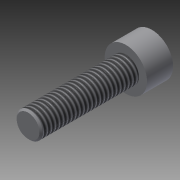
# Autodesk Inventor part: 8x30mmSHCS
Saved by Autodesk Inventor 2014 SP1 (Build 180222100, 222)
## iProperties
Created: 2013-12-15
Part Number: 8x30mmSHCS
Material: Stainless Steel
Document SubType Name: Modeling
Designer: Jack
Density: 8.08 g/cm^3
Appearance: Semi-Polished
Author: Jack
Autodesk Inventor part; units mm, degrees
ref_plane "YZ Plane" through (0, 0, 0) normal (1, 0, 0) x (0, 1, 0)
ref_plane "XZ Plane" through (0, 0, 0) normal (0, 1, 0) x (-1, 0, 0)
ref_plane "XY Plane" through (0, 0, 0) normal (0, 0, 1) x (1, 0, 0)
sketch "Sketch1" plane through (0, 0, 0) normal (0, 1, 0) x (-1, 0, 0)
  circle A0 centre (0, 0) radius 4
  dimension "d0" = 8
  constraints: 1 centre point, 1 coincident
  measures "d0" diameter of A0
extrude "Extrusion1" add sketch "Sketch1" along normal blind 30
sketch "Sketch2" plane through (0, 30, 0) normal (0, 1, 0) x (1, 0, 0)
  circle A0 centre (0, 0) radius 4 projected
  circle A1 centre (0, 0) radius 6.5
  dimension "d3" = 13
  constraints: 1 centre point, 1 coincident
  measures "d3" diameter of A1
extrude "Extrusion2" add sketch "Sketch2" along normal blind 8 contours A0 | A1
sketch "Sketch3" plane through (0, 38, 0) normal (0, 1, 0) x (1, 0, 0)
  circle A0 centre (0, 0) radius 6.5 projected
  line L0 (0, 3.4641) -> (3, 1.7321)
  line L1 (3, 1.7321) -> (3, -1.7321)
  line L2 (3, -1.7321) -> (0, -3.4641)
  line L3 (0, -3.4641) -> (-3, -1.7321)
  line L4 (-3, -1.7321) -> (-3, 1.7321)
  line L5 (-3, 1.7321) -> (0, 3.4641)
  dimension "d6" = 6
  constraints: 12 end point, 1 coincident, 1 vertical, 13 other
  measures "d6" distance between parallel lines of L1 L4
extrude "Extrusion3" cut sketch "Sketch3" against normal blind 6 contours L0 L1 L2 L3 L4 L5
thread "Thread1" size "M8x1.25" class "6g" standard "ANSI Metric M Profile" full length
chamfer "Chamfer1" distance 0.5 angle 45 1 edges at (4, 0, 0)
body "Solid1"
